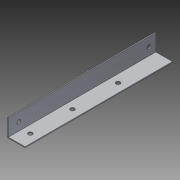
# Autodesk Inventor part: Hopper Bracing P3
Saved by Autodesk Inventor 2014 SP1 (Build 180222100, 222)
## iProperties
Created: 2013-12-16
Part Number: Hopper Bracing P3
Material: Aluminum 6061
Document SubType Name: Modeling
Designer: Moses
Mass: 8.757 g
Surface Area: 84.5036 cm^2
Volume: 3.23137 cm^3
Density: 2.71 g/cm^3
Appearance: Aluminum - Flat
Author: Moses
Autodesk Inventor part; units mm, degrees
ref_plane "YZ Plane" through (0, 0, 0) normal (1, 0, 0) x (0, 1, 0)
ref_plane "XZ Plane" through (0, 0, 0) normal (0, 1, 0) x (-1, 0, 0)
ref_plane "XY Plane" through (0, 0, 0) normal (0, 0, 1) x (1, 0, 0)
sketch "Sketch1" plane through (0, 0, 0) normal (0, 0, 1) x (1, 0, 0)
  line L0 (0, 0) -> (0, 15.875)
  line L1 (0, 15.875) -> (0.7937, 15.875)
  line L2 (0.7937, 15.875) -> (0.7938, 0.7937)
  line L3 (0.7938, 0.7937) -> (15.875, 0.7937)
  line L4 (15.875, 0.7937) -> (15.875, 0)
  line L5 (15.875, 0) -> (0, 0)
  dimension "d0" = 15.875
  dimension "d1" = 0.7937
  constraints: 12 end point, 3 horizontal, 3 vertical, 2 perpendicular
  measures "d0" distance of L0.start L0.end
  measures "d1" distance of L0.end L1.end
extrude "Extrusion1" add sketch "Sketch1" along normal blind 133.35
sketch "Sketch2" plane through (0, 0, 0) normal (0, -1, 0) x (1, 0, 0)
  line L0 (15.875, 0) -> (0, 0) projected
  line L1 (0, 133.35) -> (15.875, 133.35) projected
  line L2 (7.9375, 133.35) -> (7.9375, 0) construction
  circle A0 centre (7.9375, 120.65) radius 1.905
  circle A1 centre (7.9375, 41.275) radius 1.905
  circle A2 centre (7.9375, 82.55) radius 1.905
  dimension "d4" = 3.81
  dimension "d6" = 12.7
  dimension "d7" = 41.275
  dimension "d16" = 38.1
  constraints: 3 centre point, 3 point on line, 2 end point, 2 equal radius, 2 midpoint
  measures "d4" diameter of A0
  measures "d6" distance from line of L1 A0.centre
  measures "d7" distance of L2.end A1.centre
  measures "d16" distance of A2.centre A0.centre
extrude "Extrusion2" cut sketch "Sketch2" against normal through all
sketch "Sketch3" plane through (0, 0, 0) normal (-1, 0, 0) x (0, 0, 1)
  line L0 (0, 0) -> (0, 15.875) projected
  line L1 (133.35, 15.875) -> (133.35, 0) projected
  line L2 (0, 7.9375) -> (133.35, 7.9375) construction
  circle A0 centre (6.35, 7.9375) radius 1.905
  circle A1 centre (123.825, 7.9375) radius 1.905
  dimension "d11" = 3.81
  dimension "d12" = 9.525
  dimension "d13" = 6.35
  constraints: 2 centre point, 2 end point, 2 midpoint, 2 point on line, 1 equal radius
  measures "d11" diameter of A1
  measures "d12" distance from line of L1 A1.centre
  measures "d13" distance from line of L0 A0.centre
extrude "Extrusion3" cut sketch "Sketch3" against normal through all
body "Solid1"
